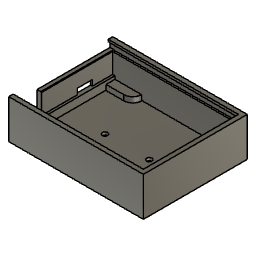
Boitier Arduino (Autodesk Fusion 360 design; units mm, degrees)
Autodesk Fusion 360 part; units mm, degrees
sketch "Esquisse1" plane through (0, 0, 0) normal (0, 0, 1) x (1, 0, 0)
  line L0 (0, 0) -> (66, 0) construction
  line L1 (66, 53) -> (0, 53) construction
  line L2 (0, 53) -> (0, 0) construction
  line L3 (66, 0) -> (66, 2) construction
  line L4 (66, 2) -> (69, 5) construction
  line L5 (69, 5) -> (69, 37) construction
  line L6 (69, 37) -> (66, 40) construction
  line L7 (66, 40) -> (66, 53) construction
  line L8 (-0.2, -0.2) -> (66.2, -0.2)
  line L9 (66.2, -0.2) -> (66.2, 1.9172)
  line L10 (66.2, 1.9172) -> (69.2, 4.9172)
  line L11 (69.2, 4.9172) -> (69.2, 37.0828)
  line L12 (69.2, 37.0828) -> (66.2, 40.0828)
  line L13 (66.2, 40.0828) -> (66.2, 53.2)
  line L14 (66.2, 53.2) -> (-0.2, 53.2)
  line L15 (-0.2, 53.2) -> (-0.2, -0.2)
  dimension "d1" = 66
  dimension "d2" = 53
  dimension "d6" = 37
  dimension "d7" = 40
  dimension "d10" = 3
  dimension "d11" = 3
  dimension "d12" = 2
  dimension "d24" = 0.2
  constraint horizontal L0
  constraint horizontal L1
  constraint vertical L2
  constraint coincident L0.start L2.end
  constraint perpendicular L1 L3
  constraint perpendicular L1 L5
  constraint vertical L7
  constraint collinear L3 L7
  measures "d1" distance of L0.start L0.end
  measures "d2" distance of L0.start L1.end
  measures "d6" vertical distance of L0.end L5.end
  measures "d7" distance of L0.end L6.end
  measures "d10" vertical distance of L3.end L4.end
  measures "d11" horizontal distance of L3.end L4.end
  measures "d12" distance of L0.end L3.end
sketch "Esquisse2" plane through (0, 0, 0) normal (0, 0, 1) x (1, 0, 0)
  circle A0 centre (14.1, 2.5) radius 1
  circle A1 centre (66.5, 35) radius 1
  circle A2 centre (66.5, 7) radius 1
  line L0 (0, 53) -> (0, 0)
  line L1 (66, 53) -> (0, 53)
  line L2 (69, 5) -> (69, 37)
  line L3 (66.5, 7) -> (66.5, 35) construction
  line L4 (0, 0) -> (66, 0) construction
  circle A3 centre (14.1, 2.5) radius 2.7
  circle A4 centre (66.5, 35) radius 2.7
  circle A5 centre (66.5, 7) radius 2.7
  line L5 (69.2, 37.0828) -> (66.2, 40.0828)
  line L6 (66.2, 40.0828) -> (66.2, 53.2)
  line L7 (66.2, 40.0828) -> (64.1305, 36.2944)
  line L8 (69.2, 4.9172) -> (69.2, 37.0828)
  line L9 (66.5, 32.3) -> (69.2, 32.3)
  arc A6 (64.1305, 36.2944) -> (66.5, 32.3) centre (66.5, 35) ccw
  line L10 (66.2, 1.9172) -> (69.2, 4.9172)
  line L11 (66.2, -0.2) -> (66.2, 1.9172)
  line L12 (66.2, 1.9172) -> (64.1305, 5.7056)
  line L13 (66.5, 9.7) -> (69.2, 9.7)
  arc A7 (66.5, 9.7) -> (64.1305, 5.7056) centre (66.5, 7) ccw
  line L14 (-0.2, -0.2) -> (66.2, -0.2)
  line L15 (16.8, 2.5) -> (16.8, -0.2)
  line L16 (11.4, 2.5) -> (11.4, -0.2)
  arc A8 (16.8, 2.5) -> (11.4, 2.5) centre (14.1, 2.5) ccw
  line L17 (0, 48) -> (10, 48)
  line L18 (10, 48) -> (10, 53) construction
  arc A9 (10, 48) -> (15, 53) centre (10, 53) ccw
  dimension "d14" = 2
  dimension "d15" = 2
  dimension "d16" = 2
  dimension "d17" = 14.1
  dimension "d20" = 2.5
  dimension "d21" = 7
  dimension "d22" = 2
  dimension "d33" = 1.7
  dimension "d34" = 2.5
  dimension "d45" = 5
  dimension "d46" = 10
  dimension "d85" = 2.7
  constraint coincident A2.centre L3.start
  constraint coincident A1.centre L3.end
  constraint vertical L3
  constraint concentric A2 A5
  constraint equal A4 A5
  constraint equal A3 A4
  constraint coincident L5.end L6.start
  constraint coincident A4 L7.end
  constraint tangent A4 L7
  constraint coincident L3 L9.start
  constraint coincident A4 L9.start
  constraint coincident L8 L9.end
  constraint tangent A4 L9
  constraint coincident L10.start L11.end
  constraint coincident A5 L12.end
  constraint tangent A5 L12
  constraint coincident L3 L13.start
  constraint coincident A5 L13.start
  constraint coincident L8 L13.end
  constraint tangent A5 L13
  constraint coincident A3 L15.start
  constraint coincident L14 L15.end
  constraint vertical L15
  constraint tangent A3 L15
  constraint coincident A3 L16.start
  constraint coincident L14 L16.end
  constraint vertical L16
  constraint tangent A3 L16
  constraint coincident A0.centre A3.centre
  constraint coincident L0 L17.start
  constraint perpendicular L0 L17
  constraint coincident L1 L18.end
  constraint perpendicular L1 L18
  constraint coincident L18.end A9.centre
  constraint equal A6 A7
  measures "d14" diameter of A0
  measures "d15" diameter of A1
  measures "d16" diameter of A2
  measures "d17" distance of A0.centre L0
  measures "d20" distance of A1.centre L2
  measures "d21" distance of A2.centre L4
  measures "d22" vertical distance of A1.centre L2.end
  measures "d34" distance of A0.centre L4
  measures "d45" distance of L1 L17
  measures "d46" distance of L17.start L17.end
  measures "d85" radius of A7
sketch "Esquisse3" plane through (0, 0, 0) normal (0, 0, 1) x (1, 0, 0)
  line L0 (-4, -1.7) -> (70.7, -1.7)
  line L1 (70.7, -1.7) -> (70.7, 54.7)
  line L2 (70.7, 54.7) -> (-4, 54.7)
  line L3 (-4, 54.7) -> (-4, -1.7)
  line L4 (-0.2, -0.2) -> (66.2, -0.2)
  line L5 (69.2, 4.9172) -> (69.2, 37.0828)
  line L6 (-5, -2.7) -> (71.7, -2.7)
  line L7 (71.7, -2.7) -> (71.7, 55.7)
  line L8 (71.7, 55.7) -> (-5, 55.7)
  line L9 (-5, 55.7) -> (-5, -2.7)
  dimension "d26" = 56.4
  dimension "d27" = 1.5
  dimension "d28" = 74.7
  dimension "d29" = 1.5
  dimension "d52" = 1
  constraint horizontal L0
  constraint vertical L1
  constraint horizontal L2
  constraint vertical L3
  measures "d26" distance of L0.start L2.end
  measures "d27" distance of L0 L4
  measures "d28" distance of L1 L3
  measures "d29" distance of L1 L5
extrude "Extrusion1" add sketch "Esquisse3" against normal blind 1.5 contours L0 L1 L2 L3
sketch "Esquisse4" plane through (0, 0, 0) normal (0, 0, 1) x (-1, 0, 0)
  line L0 (4, -54.7) -> (4, 1.7)
  line L1 (4, 1.7) -> (-70.7, 1.7)
  line L2 (-70.7, 1.7) -> (-70.7, -54.7)
  line L3 (-70.7, -54.7) -> (4, -54.7)
  line L4 (4, -54.7) -> (-70.7, -54.7)
  line L5 (-70.7, -54.7) -> (-70.7, 1.7)
  line L6 (-70.7, 1.7) -> (4, 1.7)
  line L7 (4, 1.7) -> (4, -54.7)
  line L8 (2.5, -53.2) -> (-69.2, -53.2)
  line L9 (-69.2, -53.2) -> (-69.2, 0.2)
  line L10 (-69.2, 0.2) -> (2.5, 0.2)
  line L11 (2.5, 0.2) -> (2.5, -53.2)
  line L12 (-66.2, 0.2) -> (-66.2, -1.9172)
  line L13 (-66.2, -1.9172) -> (-69.2, -4.9172)
  line L14 (-66.2, -40.0828) -> (-66.2, -53.2)
  line L15 (-69.2, -37.0828) -> (-66.2, -40.0828)
  line L16 (0.2, -53.2) -> (0.2, 0.2)
  dimension "d32" = 1.5
  constraint horizontal L4
  constraint vertical L5
  constraint horizontal L6
  constraint vertical L7
  constraint coincident L1.end L2.start
  constraint coincident L0.start L3.end
extrude "Extrusion2" add sketch "Esquisse2" along normal blind 2 contours A1 | A2 | L2 A5 A7 | A5 L8 L10 L12 | L2 A5 | L2 A5 L13 | L2 A5 L8 L13 | L2 A4 L9 | L2 A4 L8 L9 | L2 A4 A6 | L2 A4 | A4 L5 L7 L8 | A3 A8 | A3 L14 L15 | A3 L14 L16
extrude "Extrusion3" cut 3 faces at (14.0751, 0.3676, 2) (66.6102, 6.7743, 2) (66.6102, 35.2257, 2) along direction (0, 0, -1) blind 2
extrude "Extrusion4" add sketch "Esquisse2" sketch "Esquisse4" along normal blind 3 contours L2 A5 A7 | A5 L8 L10 L12 | L2 A5 | L2 A5 L13 | L2 A5 L8 L13 | L2 A4 L9 | L2 A4 L8 L9 | L2 A4 A6 | L2 A4 | A4 L5 L7 L8 | A3 A8 | A3 L14 L15 | A3 L14 L16 of sketch 2 contours L8 L9 L14 L15 | L9 L10 L12 L13
extrude "Extrusion5" add sketch "Esquisse4" along normal blind 4.5 contours L8 L10 L11 L16
extrude "Extrusion6" add sketch "Esquisse3" sketch "Esquisse4" along normal blind 20.4 and the other way up to surface of sketch 2 second end surface through (0, 0, -1.5) normal (0, 0, -1) offset 0
extrude "Extrusion7" add sketch "Esquisse2" along normal blind 3 contours L0 L1 L17 A9
sketch "Esquisse5" plane through (0, 0, -1.5) normal (0, 0, -1) x (1, 0, 0)
  line L0 (70.7, -26.5) -> (-4, -26.5) construction
  circle A0 centre (45.8, -26.5) radius 1.5
  circle A1 centre (20.9, -26.5) radius 1.5
  line L1 (20.9, -28) -> (-4, -28) construction
  line L2 (20.9, -28) -> (45.8, -28) construction
  line L3 (45.8, -28) -> (70.7, -28) construction
  line L4 (71.7, 2.7) -> (-5, 2.7)
  line L5 (-5, 2.7) -> (-5, -55.7)
  line L6 (-5, -55.7) -> (71.7, -55.7)
  line L7 (71.7, -55.7) -> (71.7, 2.7)
  dimension "d49" = 3
  constraint coincident L0 A0.centre
  constraint coincident L0 A1.centre
  constraint equal A0 A1
  constraint coincident A1 L1.start
  constraint tangent A1 L1
  constraint coincident A0 L2.end
  constraint tangent A0 L2
  constraint parallel L1 L2
  constraint tangent A0 L3
  constraint equal L1 L2
  constraint equal L2 L3
  measures "d49" diameter of A0
extrude "Extrusion8" cut sketch "Esquisse5" against normal blind 1.5 contours A0 | A1
extrude "Extrusion11" add 1 faces at (-2.5, 17.6, 9.8) along direction (1, 0, 0) blind 1
extrude "Extrusion12" cut 1 faces at (-5, 36.2333, 5.8) along direction (1, 0, 0) blind 1
sketch "Esquisse10" plane through (-1.5, 0, 0) normal (1, 0, 0) x (0, 1, 0)
  line L0 (-0.2, 4.5) -> (53.2, 4.5)
  line L1 (53.2, 4.5) -> (53.2, 20.4)
  line L2 (53.2, 20.4) -> (-0.2, 20.4)
  line L3 (-0.2, 20.4) -> (-0.2, 4.5)
  line L4 (-1.2, 18.9) -> (54.2, 18.9)
  line L5 (54.2, 18.9) -> (54.2, 15.7)
  line L6 (54.2, 15.7) -> (-1.2, 15.7)
  line L7 (-1.2, 15.7) -> (-1.2, 18.9)
  line L8 (26.5, 18.9) -> (26.5, 20.4) construction
  line L9 (-0.2, 18.9) -> (-0.2, 20.4)
  line L10 (-0.2, 20.4) -> (53.2, 20.4)
  dimension "d89" = 1.5
  dimension "d90" = 3.2
  dimension "d93" = 55.4
  constraint horizontal L4
  constraint vertical L5
  constraint horizontal L6
  constraint vertical L7
  constraint midpoint L4 L8.start
  constraint midpoint L2 L8.end
  constraint vertical L8
  constraint coincident L4 L9.start
  constraint coincident L3 L9.start
  constraint coincident L2.end L3.start
  constraint coincident L1.end L2.start
  measures "d89" distance of L8.start L8.end
  measures "d90" distance of L4 L6
  measures "d93" distance of L4.start L4.end
extrude "Extrusion17" cut sketch "Esquisse10" against normal up to surface (2.5 mm away) contours L3 L4 L6 L7 | L1 L3 L4 L6 | L1 L4 L5 L6 | L1 L2 L3 L4 L9 L10
extrude "Extrusion18" cut sketch "Esquisse10" along normal blind 71.5 contours L3 L4 L6 L7 | L1 L3 L4 L6 | L1 L4 L5 L6
sketch "Esquisse11" plane through (0, 0, 15.7) normal (0, 0, 1) x (-1, 0, 0)
  line L0 (-70, -54.2) -> (4, -54.2)
  line L1 (4, -54.2) -> (4, 1.2)
  line L2 (4, 1.2) -> (-70, 1.2)
  line L3 (-70, 1.2) -> (-70, -54.2)
  line L4 (1.5, -53.2) -> (-69.2, -53.2)
  line L5 (-69.2, -53.2) -> (-69.2, 0.2)
  line L6 (-69.2, 0.2) -> (1.5, 0.2)
  line L7 (1.5, 0.2) -> (1.5, -53.2)
  line L8 (1.9, -54.2) -> (1.9, 1.2)
  dimension "d98" = 71.9
  constraint coincident L0 L8.start
  constraint coincident L2 L8.end
  constraint perpendicular L2 L8
  measures "d98" distance of L3 L8
extrude "Extrusion19" add sketch "Esquisse11" along normal blind 0.2 contours L0 L1 L2 L8
sketch "Esquisse7" plane through (-1.5, 0, 0) normal (1, 0, 0) x (0, 1, 0)
  line L0 (-0.2, 15.7) -> (-0.2, 4.5)
  line L1 (-0.2, 4.5) -> (53.2, 4.5)
  line L2 (53.2, 4.5) -> (53.2, 15.7)
  line L3 (3.8, 4.5) -> (13.2, 4.5)
  line L4 (13.2, 4.5) -> (13.2, 15.9)
  line L5 (13.2, 15.9) -> (3.8, 15.9)
  line L6 (3.8, 15.9) -> (3.8, 4.5)
  line L7 (33.4, 4.5) -> (41.8, 4.5)
  line L8 (41.8, 4.5) -> (41.8, 7.7)
  line L9 (41.8, 7.7) -> (33.4, 7.7)
  line L10 (33.4, 7.7) -> (33.4, 4.5)
  line L11 (53.2, 15.7) -> (-0.2, 15.7)
  dimension "d66" = 9.4
  dimension "d67" = 11.4
  dimension "d68" = 4
  dimension "d71" = 8.4
  dimension "d72" = 3.2
  dimension "d73" = 11.4
  constraint horizontal L3
  constraint vertical L4
  constraint horizontal L5
  constraint vertical L6
  constraint coincident L1 L3.start
  constraint horizontal L7
  constraint vertical L8
  constraint horizontal L9
  constraint vertical L10
  constraint coincident L1 L7.start
  measures "d66" distance of L3.start L3.end
  measures "d67" distance of L3.start L5.end
  measures "d68" distance of L0.end L6
  measures "d71" distance of L7.start L7.end
  measures "d72" distance of L7.start L9.end
  measures "d73" distance of L2 L8
extrude "Extrusion14" cut sketch "Esquisse7" against normal blind 2.5 contours L1 L3 L4 L6 L11 | L4 L5 L6 L11 | L1 L7 L8 L9 L10
sketch "Esquisse8" plane through (-4, 0, 0) normal (-1, 0, 0) x (0, -1, 0)
  line L0 (-3.8, 4.5) -> (-13.2, 4.5)
  line L1 (-13.2, 4.5) -> (-13.2, 15.9)
  line L2 (-3.8, 15.9) -> (-3.8, 4.5)
  line L3 (-33.4, 4.5) -> (-41.8, 4.5)
  line L4 (-41.8, 4.5) -> (-41.8, 7.7)
  line L5 (-41.8, 7.7) -> (-33.4, 7.7)
  line L6 (-33.4, 7.7) -> (-33.4, 4.5)
  line L7 (-53.2, 20.4) -> (-55.7, 20.4)
  line L8 (-55.7, -1.5) -> (2.7, -1.5)
  line L9 (-31.9, 3) -> (-43.3, 3)
  line L10 (-43.3, 3) -> (-43.3, 9.2)
  line L11 (-43.3, 9.2) -> (-31.9, 9.2)
  line L12 (-31.9, 9.2) -> (-31.9, 3)
  line L13 (2.7, -1.5) -> (2.7, 20.4)
  line L14 (-55.7, 20.4) -> (-55.7, -1.5)
  line L15 (-13.2, 15.9) -> (-54.2, 15.9)
  line L16 (-54.2, 15.9) -> (-54.2, 18.9)
  line L17 (-54.2, 18.9) -> (-53.2, 18.9)
  line L18 (-53.2, 18.9) -> (-53.2, 20.4)
  line L19 (2.7, 20.4) -> (0.2, 20.4)
  line L20 (0.2, 20.4) -> (0.2, 18.9)
  line L21 (0.2, 18.9) -> (1.2, 18.9)
  line L22 (1.2, 18.9) -> (1.2, 15.9)
  line L23 (1.2, 15.9) -> (-3.8, 15.9)
  dimension "d79" = -1.5
extrude "Extrusion16" cut sketch "Esquisse8" against normal blind 1.5 contours L9 L10 L11 L12
chamfer "Chanfrein1" distance 1.5 angle 45 4 edges at (-4, 31.9, 6.1) (-4, 37.6, 9.2) (-4, 43.3, 6.1) (-4, 37.6, 3)
draft "Dépouille1" angle 0.2 neutral plane through (70, 0, 0) pull (-1, 0, 0) 1 faces at (45.0667, -0.8667, 18.9)
equation "d1 = longArduino"
equation "d2 = largArduino"
equation "longArduino = 66 mm"
equation "largArduino = 53 mm"
equation "d6 = longEncoche - largEncoche"
equation "d7 = longEncoche"
equation "longEncoche = 40 mm"
equation "largEncoche = 3 mm"
equation "d10 = largEncoche"
equation "d11 = largEncoche"
equation "percageArduino = 2 mm"
equation "d14 = percageArduino"
equation "d15 = percageArduino"
equation "d16 = percageArduino"
equation "decalagePercage = 2.5 mm"
equation "d20 = decalagePercage"
equation "decalageImpression = 0.2 mm"
equation "d24 = decalageImpression"
equation "epaisseurBoitier = 1.5 mm"
equation "d26 = largArduino + ( epaisseurBoitier + decalageImpression ) * 2"
equation "d27 = epaisseurBoitier"
equation "d28 = longArduino + largEncoche + epaisseurBoitier + decalageImpression + 4 mm"
equation "d29 = epaisseurBoitier"
equation "d33 = epaisseurBoitier + decalageImpression"
equation "d34 = decalagePercage"
equation "d41 = 3 mm + 1.5 mm"
equation "d43 = 20 mm - 1.3 mm + epaisseurBoitier + decalageImpression"
equation "largPriseDC = 9 mm"
equation "longPriseDC = 11 mm"
equation "d66 = largPriseDC + decalageImpression * 2"
equation "d67 = longPriseDC + decalageImpression * 2"
equation "largPriseUSB = 3 mm"
equation "longPriseUSB = 8 mm"
equation "d71 = longPriseUSB + decalageImpression * 2"
equation "d72 = largPriseUSB + decalageImpression"
equation "epaisseurPlexi = 3 mm"
equation "d89 = epaisseurBoitier"
equation "d90 = epaisseurPlexi + decalageImpression"
equation "largeurPlexi = 55 mm"
equation "longueurPlexi = 71.5 mm"
equation "d93 = largeurPlexi + decalageImpression * 2"
equation "d96 = longueurPlexi"
equation "d98 = longueurPlexi + decalageImpression * 2"
equation "d99 = decalageImpression"
